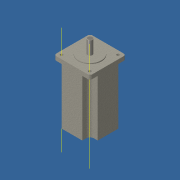
# Autodesk Inventor part: Nema24 - L100
Saved by Autodesk Inventor 2016 SP1 (Build 200210100, 210)
## iProperties
Created: 2015-08-24
Part Number: Nema24 - L100
Material: Stahl
Document SubType Name: Modeling
Designer: 4ndreas
Density: 5.2618 g/cm^3
Appearance: Stahl - Guss
Mass: 1600 g
Surface Area: 316.212 cm^2
Volume: 305.128 cm^3
Description: http://www.omc-stepperonline.com/dual-shaft-cnc-stepper-motor-nema-24-100mm-4nm566-ozin-24hs393008d-p-388.html
Author: 4ndreas
Autodesk Inventor part; units mm, degrees
ref_plane "YZ Plane" through (0, 0, 0) normal (1, 0, 0) x (0, 1, 0)
ref_plane "XZ Plane" through (0, 0, 0) normal (0, 1, 0) x (-1, 0, 0)
ref_plane "XY Plane" through (0, 0, 0) normal (0, 0, 1) x (1, 0, 0)
sketch "Skizze1" plane through (0, 0, 0) normal (0, 0, 1) x (1, 0, 0)
  line L0 (-26, -30) -> (26, -30)
  line L1 (30, -26) -> (30, 26)
  line L2 (26, 30) -> (-26, 30)
  line L3 (-30, 26) -> (-30, -26)
  line L4 (-30, -30) -> (30, 30) construction
  line L5 (30, -30) -> (-30, 30) construction
  arc A0 (30, 26) -> (26, 30) centre (26, 26) ccw
  arc A1 (26, -30) -> (30, -26) centre (26, -26) ccw
  arc A2 (-30, -26) -> (-26, -30) centre (-26, -26) ccw
  arc A3 (-26, 30) -> (-30, 26) centre (-26, 26) ccw
  point P0 (0, 0)
  dimension "d0" = 4
  dimension "d1" = 60
  constraints: 12 end point, 8 point on circle, 8 point on line, 8 tangent, 4 centre point, 3 equal radius, 2 midpoint, 2 parallel, 2 perpendicular, 1 horizontal
  measures "d0" radius of A0
  measures "d1" distance between parallel lines of L0 L2
extrude "Extrusion1" add sketch "Skizze1" against normal blind 100
sketch "Skizze2" plane through (0, 0, 0) normal (0, 0, 1) x (1, 0, 0)
  circle A0 centre (0, 0) radius 19.05
  dimension "d4" = 38.1
  constraints: 1 centre point, 1 coincident
  measures "d4" diameter of A0
extrude "Extrusion2" add sketch "Skizze2" along normal blind 1.6
sketch "Skizze4" plane through (0, 0, 0) normal (0, 0, 1) x (1, 0, 0)
  circle A0 centre (0, 0) radius 19.05 projected
  line L0 (30, 26) -> (30, -26) projected
  arc A1 (30, 26) -> (26, 30) centre (26, 26) ccw projected
  line L1 (-26, 30) -> (26, 30) projected
  arc A2 (-26, 30) -> (-30, 26) centre (-26, 26) ccw projected
  line L2 (-30, -26) -> (-30, 26) projected
  arc A3 (-30, -26) -> (-26, -30) centre (-26, -26) ccw projected
  line L3 (26, -30) -> (-26, -30) projected
  arc A4 (26, -30) -> (30, -26) centre (26, -26) ccw projected
  line L4 (26, -26) -> (-26, 26) construction
  line L5 (-23.57, 23.57) -> (23.57, 23.57) construction
  line L6 (23.57, 23.57) -> (23.57, -23.57) construction
  line L7 (23.57, -23.57) -> (-23.57, -23.57) construction
  line L8 (-23.57, -23.57) -> (-23.57, 23.57) construction
  line L9 (-23.57, 23.57) -> (23.57, -23.57) construction
  line L10 (23.57, 23.57) -> (-23.57, -23.57) construction
  dimension "d15" = 47.14
  constraints: 14 end point, 2 midpoint, 2 parallel, 1 horizontal, 1 perpendicular, 1 point on line
  measures "d15" distance between parallel lines of L8 L6
hole "Bohrung1" at (23.57, 23.57, 0) at (-23.57, 23.57, 0) at (-23.57, -23.57, 0) at (23.57, -23.57, 0) direction (0, 0, -1) diameter 4.5 end through all
sketch "Skizze5" plane through (0, 0, 1.6) normal (0, 0, 1) x (1, 0, 0)
  circle A0 centre (0, 0) radius 4
  dimension "d23" = 8
  constraints: 1 centre point, 1 coincident
  measures "d23" diameter of A0
extrude "Extrusion4" add sketch "Skizze5" along normal blind 22.4
sketch "Skizze7" plane through (0, 0, -100) normal (0, 0, -1) x (-1, 0, 0)
  circle A0 centre (23.57, -23.57) radius 2.25 projected
  circle A1 centre (-23.57, 23.57) radius 2.25 projected
  circle A2 centre (23.57, 23.57) radius 2.25 projected
  circle A3 centre (-23.57, -23.57) radius 2.25 projected
  line L0 (-30, 26) -> (-30, -26) projected
  arc A4 (-30, -26) -> (-26, -30) centre (-26, -26) ccw projected
  line L1 (-26, -30) -> (26, -30) projected
  arc A5 (26, -30) -> (30, -26) centre (26, -26) ccw projected
  line L2 (30, -26) -> (30, 26) projected
  arc A6 (30, 26) -> (26, 30) centre (26, 26) ccw projected
  line L3 (26, 30) -> (-26, 30) projected
  arc A7 (-26, 30) -> (-30, 26) centre (-26, 26) ccw projected
  circle A8 centre (23.57, -23.57) radius 6.43 construction
  line L4 (30, -26) -> (30, 26) projected
  line L5 (30, -17.14) -> (23.57, -17.14)
  line L6 (-26, -30) -> (26, -30) projected
  line L7 (17.14, -30) -> (17.14, -23.57)
  arc A9 (23.57, -17.14) -> (17.14, -23.57) centre (23.57, -23.57) ccw
  arc A10 (-17.14, -23.57) -> (-23.57, -17.14) centre (-23.57, -23.57) ccw
  arc A11 (17.2019, 24.4599) -> (23.57, 17.14) centre (23.57, 23.57) ccw
  arc A12 (-23.57, 17.14) -> (-17.14, 23.57) centre (-23.57, 23.57) ccw
  line L8 (23.57, 17.14) -> (30, 17.14)
  line L9 (17.14, 23.57) -> (17.14, 30)
  line L10 (26, 30) -> (-26, 30) projected
  line L11 (-17.14, 23.57) -> (-17.14, 30)
  line L12 (-23.57, 17.14) -> (-30, 17.14)
  line L13 (-23.57, -17.14) -> (-30, -17.14)
  line L14 (-17.14, -23.57) -> (-17.14, -30)
  point P0 (0, 0)
  constraints: 16 end point, 11 point on circle, 9 point on line, 9 tangent, 5 centre point, 5 coincident, 4 perpendicular, 3 equal radius, 2 equal length, 2 parallel
extrude "Extrusion6" cut sketch "Skizze7" against normal blind 93.2 contours A7 L3 L11 A12 L12 L0 | L13 A10 L14 L1 A4 L0 | L3 A6 L2 L8 A11 L9 | L7 A9 L5 L2 A5 L1
sketch "Skizze8" plane through (0, 0, -100) normal (0, 0, -1) x (-1, 0, 0)
  circle A0 centre (23.57, -23.57) radius 2.25 construction
  circle A1 centre (-23.57, 23.57) radius 2.25 construction
  circle A2 centre (23.57, 23.57) radius 2.25 construction
  circle A3 centre (-23.57, -23.57) radius 2.25 construction
  circle A4 centre (0, 0) radius 19.05 construction
  line L0 (-30, 26) -> (-30, -26) construction
  arc A5 (-26, 30) -> (-30, 26) centre (-26, 26) ccw construction
  line L1 (26, 30) -> (-26, 30) construction
  arc A6 (30, 26) -> (26, 30) centre (26, 26) ccw construction
  line L2 (30, -26) -> (30, 26) construction
  arc A7 (26, -30) -> (30, -26) centre (26, -26) ccw construction
  line L3 (-26, -30) -> (26, -30) construction
  arc A8 (-30, -26) -> (-26, -30) centre (-26, -26) ccw construction
  circle A9 centre (0, 0) radius 42.4264 construction
  line L4 (30, 30) -> (-30, 30) construction
  line L5 (-30, 30) -> (-30, -30) construction
  line L6 (-30, -30) -> (30, -30) construction
  line L7 (30, -30) -> (30, 30) construction
  line L8 (30, 30) -> (-30, -30) construction
  line L9 (-30, 30) -> (30, -30) construction
  line L10 (-17.14, -30) -> (17.14, -30) construction
  line L11 (-30, 17.14) -> (-30, -17.14) construction
  constraints: 12 end point, 2 collinear, 2 midpoint, 2 parallel, 1 coincident, 1 horizontal, 1 perpendicular, 3 other
sketch "Skizze9" plane through (0, 0, -100) normal (0, 0, -1) x (-1, 0, 0)
  circle A0 centre (0, 0) radius 4 projected
extrude "Extrusion7" add sketch "Skizze9" along normal blind 15
chamfer "Fase1" distance 0.5 angle 45 2 edges at (4, 0, -115) (-4, 0, 24)
equation "\"d1\" = breite"
equation "\"d2\" = Laenge"
equation "\"d4\" = fit"
equation "\"d5\" = fit_l"
equation "\"d15\" = lochabstand"
equation "\"d16\" = bohrung_d"
equation "\"d23\" = schaft_d"
equation "\"d24\" = schaft_l"
equation "\"d28\" = Laenge - Mount_l"
equation "\"breite\" = 60"
equation "\"lochabstand\" = 47.14"
equation "\"schaft_d\" = 8"
equation "\"fit\" = 38.1"
equation "\"fit_l\" = 1.6"
equation "\"Mount_l\" = 6.8"
equation "\"Laenge\" = 100"
equation "\"bohrung_d\" = 4.5"
equation "\"schaft_l\" = 22.4"
